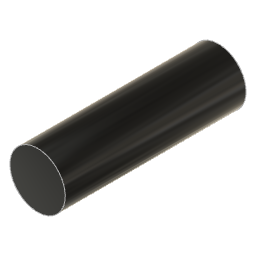
_Power Cell.fb1e0a0f-94d6-485b-973a-2a5ea20c2e34 (Autodesk Fusion 360 design; units mm, degrees)
Autodesk Fusion 360 part; units mm, degrees
sketch "Sketch1" plane through (0, 0, 0) normal (0, 1, 0) x (1, 0, 0)
  circle A0 centre (12.7, -12.7) radius 16.51
  dimension "d1" = 33.02
  measures "d1" diameter of A0
extrude "Extrude1" add sketch "Sketch1" along normal blind 107.95
